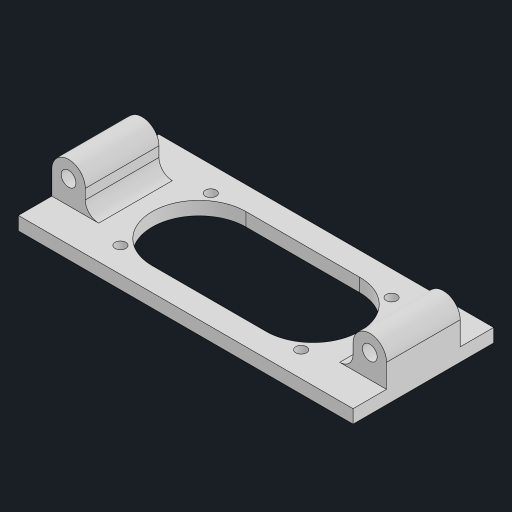
# Autodesk Inventor part: Ultrasonic_holderV2
Saved by Autodesk Inventor 2023 (Build 270158000, 158)
## iProperties
Created: 2022-06-21
Part Number: Ultrasonic_holderV2
Material: 一般
Document SubType Name: Modeling
Designer: legot
Density: 1 g/cm^3
Appearance: 既定
Author: legot
Autodesk Inventor part; units mm, degrees
ref_plane "YZ Plane" through (0, 0, 0) normal (1, 0, 0) x (0, 1, 0)
ref_plane "XZ Plane" through (0, 0, 0) normal (0, 1, 0) x (-1, 0, 0)
ref_plane "XY Plane" through (0, 0, 0) normal (0, 0, 1) x (1, 0, 0)
sketch "スケッチ1" plane through (0, 0, 0) normal (0, 1, 0) x (-1, 0, 0)
  line L0 (0, 6.75) -> (-13.5, 6.75) construction
  line L1 (-13.5, 6.75) -> (-13.5, -6.75) construction
  line L2 (-13.5, -6.75) -> (0, -6.75) construction
  line L3 (0, -6.75) -> (0, 6.75) construction
  circle A0 centre (-8.5, 0) radius 7
  line L4 (0, 10.5) -> (-25, 10.5)
  line L5 (-25, 10.5) -> (-25, -10.5)
  line L6 (-25, -10.5) -> (0, -10.5)
  line L7 (0, -10.5) -> (0, 10.5)
  line L8 (-25, -6.5) -> (-25, 10.5)
  line L9 (0, 7) -> (-8.5, 7)
  line L10 (0, -7) -> (-8.5, -7)
  point P0 (0, 0)
  point P1 (0, 0)
  dimension "d0" = 13.5
  dimension "d1" = 13.5
  dimension "d2" = 8.5
  dimension "d3" = 14
  dimension "d4" = 21
  dimension "d5" = 25
  constraints: 22 end point, 4 parallel, 3 coincident, 3 horizontal, 3 perpendicular, 2 midpoint, 2 point on circle, 2 point on line, 2 tangent, 1 centre point, 1 horizontal alignment
  measures "d0" distance of L2.end L0.start
  measures "d1" distance of L0.start L0.end
  measures "d2" distance of A0.centre point (0, 0)
  measures "d3" diameter of A0
  measures "d4" distance of L6.end L4.start
  measures "d5" distance of L5.end L6.end
extrude "押し出し1" add sketch "スケッチ1" along normal blind 2 contours A0 L10 L7 L6 L5 L4 L9
hole "穴1" at (13.5, 0, -6.75) at (13.5, 0, 6.75) direction (0, 1, 0) diameter 1.6 end through all clearance for "Flat Head Machine Screw (82)" size "#0" standard "Ansi Unified Screw Threads"
sketch "スケッチ3" plane through (0, 0, 0) normal (0, 0, 1) x (1, 0, 0)
  line L0 (25, 0) -> (0, 0) projected
  line L1 (0, 0) -> (0, 2) projected
  line L2 (25, 2) -> (0, 2) projected
  line L3 (25, 0) -> (25, 2) projected
  line L4 (25, 2) -> (25, 9)
  line L5 (25, 9) -> (20, 9)
  line L6 (20, 9) -> (20, 2)
  circle A0 centre (22.5, 5.5) radius 1.1
  circle A1 centre (22.5, 5.5) radius 3.5 construction
  arc A2 (25, 5.5) -> (20, 5.5) centre (22.5, 5.5) ccw
  arc A3 (20, 5.5) -> (25, 5.5) centre (22.5, 5.5) ccw construction
  point P0 (0, 0)
  point P1 (22.5, 9)
  dimension "d27" = 7
  dimension "d29" = 2.2
  dimension "d30" = 5
  constraints: 6 end point, 4 centre point, 4 point on circle, 3 midpoint, 3 tangent, 2 coincident, 2 perpendicular, 1 point on line, 1 vertical, 1 vertical alignment
  measures "d27" diameter of A1
  measures "d29" diameter of A0
  measures "d30" diameter of A2
extrude "押し出し3" add sketch "スケッチ3" along normal mid plane 11 contours L2 L6 A2 L4
fillet "フィレット2" radius 2 1 edges at (20, 2, 0)
mirror "ミラー2" about plane through (0, 0, 0) normal (1, 0, 0) of "押し出し1", "穴1", "押し出し3", "フィレット2"
